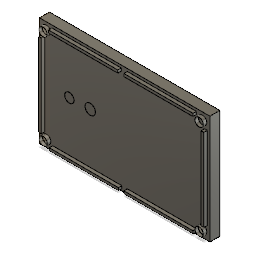
arduino_lid v1 (Autodesk Fusion 360 design; units mm, degrees)
Autodesk Fusion 360 part; units mm, degrees
sketch "Sketch1" plane through (0, 0, 0) normal (0, 0, 1) x (1, 0, 0)
  line L0 (63.5, -40.64) -> (-63.5, -40.64)
  line L1 (-63.5, -40.64) -> (-63.5, 40.64)
  line L2 (-63.5, 40.64) -> (63.5, 40.64)
  line L3 (63.5, 40.64) -> (63.5, -40.64)
  line L4 (63.5, -40.64) -> (-63.5, 40.64) construction
  line L5 (-63.5, -40.64) -> (63.5, 40.64) construction
  dimension "d1" = 127
  dimension "d2" = 81.28
extrude "Extrude1" add sketch "Sketch1" along normal blind 7.62
sketch "Sketch2" plane through (0, 0, 7.62) normal (0, 0, 1) x (1, 0, 0)
  line L0 (63.5, 40.64) -> (-63.5, 40.64)
  line L1 (-63.5, 40.64) -> (-63.5, -40.64)
  line L2 (-63.5, -40.64) -> (63.5, -40.64)
  line L3 (63.5, -40.64) -> (63.5, 40.64)
  circle A0 centre (-58.2936, 35.3456) radius 3.175
  circle A1 centre (58.0185, 35.3182) radius 3.175
  circle A2 centre (-58.0728, -35.0014) radius 3.175
  circle A3 centre (58.0185, -35.2572) radius 3.175
  dimension "d5" = 6.35
  dimension "d6" = 6.35
  dimension "d7" = 6.35
  dimension "d8" = 6.35
  measures "d5" diameter of A0
  measures "d6" diameter of A1
  measures "d7" diameter of A2
  measures "d8" diameter of A3
extrude "Extrude2" add sketch "Sketch2" along normal blind 2.54 contours A0 | A1 | A2 | A3
shell "Shell1" thickness 0.1 removed faces 4 at (57.2005, -34.4297, 10.16) at (-58.9534, 34.5182, 10.16) at (57.2005, 36.1456, 10.16) at (-58.1519, -34.2237, 10.16)
box "BoxPrimitive1" add length 2.032 width 51.6529 height 2.54 placed x (0, -1, 0) y (1, 0, 0) z (0, 0, 1) at (-54.1348, 38.6952, 7.62)
box "BoxPrimitive2" add length 2.032 width 51.4096 height 2.54 placed x (0, -1, 0) y (1, 0, 0) z (0, 0, 1) at (2.0106, 38.6952, 7.62)
box "BoxPrimitive3" add length 61.8009 width 2.032 height 2.54 placed x (0, -1, 0) y (1, 0, 0) z (0, 0, 1) at (-61.5167, 30.8433, 7.62)
box "BoxPrimitive4" add length 2.032 width 51.4096 height 2.54 placed x (0, -1, 0) y (1, 0, 0) z (0, 0, 1) at (-53.4602, -36.9342, 7.62)
box "BoxPrimitive5" add length 2.032 width 51.4096 height 2.54 placed x (0, -1, 0) y (1, 0, 0) z (0, 0, 1) at (2.0369, -36.9342, 7.62)
sketch "Sketch8" plane through (-63.4, 0, 0) normal (1, 0, 0) x (0, 0, -1)
  line L0 (-0.1, -40.54) -> (-0.1, 40.54)
  line L1 (-0.1, 40.54) -> (-7.52, 40.54)
  line L2 (-7.52, 40.54) -> (-7.52, -40.54)
  line L3 (-7.52, -40.54) -> (-0.1, -40.54)
sketch "Sketch9" plane through (0, 0, 7.62) normal (0, 0, 1) x (1, 0, 0)
  line L0 (2.0369, -38.9662) -> (2.0369, -36.9342)
  line L1 (2.0369, -36.9342) -> (53.4465, -36.9342)
  line L2 (53.4465, -36.9342) -> (53.4465, -38.9662)
  line L3 (53.4465, -38.9662) -> (2.0369, -38.9662)
  line L4 (-53.4602, -38.9662) -> (-53.4602, -36.9342)
  line L5 (-53.4602, -36.9342) -> (-2.0506, -36.9342)
  line L6 (-2.0506, -36.9342) -> (-2.0506, -38.9662)
  line L7 (-2.0506, -38.9662) -> (-53.4602, -38.9662)
  line L8 (-61.5167, -30.9576) -> (-61.5167, 30.8433)
  line L9 (-61.5167, 30.8433) -> (-59.4847, 30.8433)
  line L10 (-59.4847, 30.8433) -> (-59.4847, -30.9576)
  line L11 (-59.4847, -30.9576) -> (-61.5167, -30.9576)
  line L12 (2.0106, 36.6632) -> (2.0106, 38.6952)
  line L13 (2.0106, 38.6952) -> (53.4202, 38.6952)
  line L14 (53.4202, 38.6952) -> (53.4202, 36.6632)
  line L15 (53.4202, 36.6632) -> (2.0106, 36.6632)
  line L16 (-54.1348, 36.6632) -> (-54.1348, 38.6952)
  line L17 (-54.1348, 38.6952) -> (-2.4819, 38.6952)
  line L18 (-2.4819, 38.6952) -> (-2.4819, 36.6632)
  line L19 (-2.4819, 36.6632) -> (-54.1348, 36.6632)
  circle A0 centre (-58.0728, -35.0014) radius 3.175
  circle A1 centre (-58.2936, 35.3456) radius 3.175
  circle A2 centre (58.0185, -35.2572) radius 3.175
  circle A3 centre (58.0185, 35.3182) radius 3.175
  line L20 (63.5, 40.64) -> (-63.5, 40.64)
  line L21 (-63.5, 40.64) -> (-63.5, -40.64)
  line L22 (-63.5, -40.64) -> (63.5, -40.64)
  line L23 (63.5, -40.64) -> (63.5, 40.64)
  line L24 (63.5, -21.6408) -> (61.5188, -21.6408)
  circle A4 centre (-41.1386, 0.1686) radius 3.5
  circle A5 centre (-25.6273, 0.5058) radius 3.9
  dimension "d37" = 1.9812
  dimension "d43" = 7
  dimension "d44" = 7.8
  measures "d43" diameter of A4
  measures "d44" diameter of A5
extrude "Extrude3" cut sketch "Sketch9" against normal blind 127 contours A4 | A5
box "BoxPrimitive6" add length 61.2943 width 2.032 height 2.54 placed x (0, 1, 0) y (-1, 0, 0) z (0, 0, 1) at (61.5188, -30.7792, 7.62)
